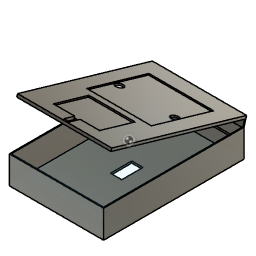
Round2-CAD (Autodesk Fusion 360 design; units mm, degrees)
Autodesk Fusion 360 part; units mm, degrees
sketch "Sketch6" plane through (0, 0, 0) normal (0, 0, 1) x (1, 0, 0)
  line L0 (0, 0) -> (0, 152)
  line L1 (0, 152) -> (102, 152)
  line L2 (102, 152) -> (102, 0)
  line L3 (102, 0) -> (0, 0)
  line L4 (375, 0) -> (375, 150)
  line L5 (375, 150) -> (475, 150)
  line L6 (475, 150) -> (475, 0)
  line L7 (475, 0) -> (375, 0)
  dimension "d16" = 152
  dimension "d17" = 102
  dimension "d89" = 150
  dimension "d90" = 100
  constraint coincident L0.start L3.end
  constraint vertical L0
  constraint perpendicular L0 L1
  constraint perpendicular L1 L2
  constraint perpendicular L0 L3
  constraint vertical L4
  constraint perpendicular L4 L5
  constraint perpendicular L5 L6
  constraint perpendicular L4 L7
  measures "d16" distance of L0.start L0.end
  measures "d17" distance of L0.end L1.end
  measures "d89" distance of L4.start L4.end
  measures "d90" distance of L4.end L5.end
extrude "Extrude2" add sketch "Sketch6" along normal blind 30 contours L0 L1 L2 L3 picked at (34, 101.333333)
shell "Shell1" thickness 2 removed faces 1 at (34, 101.333333, 30)
sketch "Sketch7" plane through (0, 0, 0) normal (0, 0, -1) x (1, 0, 0)
  line L0 (102, -152) -> (102, 0)
  line L1 (102, 0) -> (0, 0)
  line L2 (0, 0) -> (0, -152)
  line L3 (0, -152) -> (102, -152)
  line L4 (57.1, -64.5) -> (44.9, -64.5)
  line L5 (57.1, -87.5) -> (57.1, -64.5)
  line L6 (57.1, -64.5) -> (44.9, -64.5)
  line L7 (44.9, -64.5) -> (44.9, -87.5)
  line L8 (44.9, -87.5) -> (57.1, -87.5)
  line L9 (57.1, -87.5) -> (57.1, -64.5)
  constraint vertical L5
  constraint horizontal L6
  constraint vertical L7
  constraint horizontal L8
  constraint vertical L9
extrude "Extrude3" cut sketch "Sketch7" against normal blind 30 contours L4 L5 L6 L7 L8 L9 picked at (48.966667, -72.166667)
sketch "Sketch10" plane through (0, 0, 0) normal (-1, 0, 0) x (0, -1, 0)
  line L0 (-152, 0) -> (0, 0)
  line L1 (0, 0) -> (0, 30)
  line L2 (0, 30) -> (-152, 30)
  line L3 (-152, 30) -> (-152, 0)
  line L4 (-152, 30) -> (-6.038555, 72.417643)
  line L5 (-6.038555, 72.417643) -> (-5.201364, 69.536825)
  line L6 (-5.201364, 69.536825) -> (-151.16281, 27.119182)
  line L7 (-151.16281, 27.119182) -> (-152, 30)
  dimension "d30" = 152
  dimension "d31" = 3
  constraint perpendicular L4 L5
  constraint parallel L4 L6
  constraint parallel L5 L7
  constraint coincident L2.end L3.start
extrude "Extrude4" add sketch "Sketch10" against normal blind 102 contours L2 L4 L5 L6 picked at (-99.76277, 44.139214)
sketch "Sketch11" plane through (0, 19.876523, 68.396211) normal (0, 0.279063, 0.960273) x (-1, 0, 0)
  line L0 (0, -137.589542) -> (0, 14.410458)
  line L1 (0, 14.410458) -> (-102, 14.410458)
  line L2 (-102, 14.410458) -> (-102, -137.589542)
  line L3 (-102, -137.589542) -> (0, -137.589542)
  line L4 (-85.31414, -47.669713, 3.681927) -> (-15.31414, -47.669713, 3.681927)
  line L5 (-15.31414, -47.669713, 3.681927) -> (-15.31414, -117.669713, 3.681927)
  line L6 (-15.31414, -117.669713, 3.681927) -> (-85.31414, -117.669713, 3.681927)
  line L7 (-85.31414, -117.669713, 3.681927) -> (-85.31414, -47.669713, 3.681927)
  line L8 (-85.31414, -47.669713, 3.681927) -> (-15.31414, -117.669713, 3.681927) construction
  line L9 (-15.31414, -47.669713, 3.681927) -> (-85.31414, -117.669713, 3.681927) construction
  circle A0 centre (-80, -80) radius 3.5
  circle A1 centre (-20, -80) radius 3.5
  point P0 (-50.31414, -82.669713)
  dimension "d34" = 70
  dimension "d35" = 70
  dimension "d38" = 7
  dimension "d39" = 7
  measures "d38" diameter of A0
  measures "d39" diameter of A1
extrude "Extrude5" cut sketch "Sketch11" against normal blind 5 contours L4 L5 L6 L7 in plane through (0, 20.904007, 71.931839) normal (0, 0.27906344, 0.96027267) picked at (61.980806, 89.086291, 52.117485)
extrude "Extrude6" cut sketch "Sketch11" against normal blind 10 draft 30 contours A0 | A1 picked at (-81.114835, -79.656119) picked at (-20.259608, -78.862584)
sketch "Sketch12" plane through (0, 19.876523, 68.396211) normal (0, 0.279063, 0.960273) x (-1, 0, 0)
  line L0 (-15.31414, -47.669713) -> (-15.31414, -117.669713)
  line L1 (-15.31414, -117.669713) -> (-85.31414, -117.669713)
  line L2 (-85.31414, -117.669713) -> (-85.31414, -47.669713)
  line L3 (-85.31414, -47.669713) -> (-15.31414, -47.669713)
  line L4 (0, -137.589542) -> (0, 14.410458)
  line L5 (0, 14.410458) -> (-102, 14.410458)
  line L6 (-102, 14.410458) -> (-102, -137.589542)
  line L7 (-102, -137.589542) -> (0, -137.589542)
  line L8 (-50, 0) -> (-75, 0) construction
  line L9 (-75, 0) -> (-25, 0)
  line L10 (-25, 0) -> (-25, -40)
  line L11 (-25, -40) -> (-75, -40)
  line L12 (-75, -40) -> (-75, 0)
  dimension "d43" = 50
  dimension "d44" = 40
  constraint horizontal L9
  constraint vertical L10
  constraint horizontal L11
  constraint vertical L12
  measures "d43" distance of L8.end L9.end
  measures "d44" distance of L8.end L11.end
extrude "Extrude7" cut sketch "Sketch12" against normal blind 0.5 contours L9 L10 L11 L12 picked at (-58.333333, -13.333333)
extrude "Extrude8" cut 1 faces at (58.333333, 45.344263, 60.474383) along direction (0, -0.27906344, -0.96027267) blind 1
sketch "Sketch15" plane through (0, 19.876523, 68.396211) normal (0, 0.279063, 0.960273) x (-1, 0, 0)
  line L0 (-25, 0) -> (-25, -40)
  line L1 (-25, -40) -> (-75, -40)
  line L2 (-75, -40) -> (-75, 0)
  line L3 (-75, 0) -> (-25, 0)
  line L4 (-15.31414, -47.669713) -> (-15.31414, -117.669713)
  line L5 (-15.31414, -117.669713) -> (-85.31414, -117.669713)
  line L6 (-85.31414, -117.669713) -> (-85.31414, -47.669713)
  line L7 (-85.31414, -47.669713) -> (-15.31414, -47.669713)
  line L8 (0, -137.589542) -> (0, 14.410458)
  line L9 (0, 14.410458) -> (-102, 14.410458)
  line L10 (-102, 14.410458) -> (-102, -137.589542)
  line L11 (-102, -137.589542) -> (0, -137.589542)
  line L12 (-51, 0) -> (-54, 0)
  line L13 (-54, 0) -> (-48, 0)
  line L14 (-48, 0) -> (-48, 12)
  line L15 (-48, 12) -> (-54, 12)
  line L16 (-54, 12) -> (-54, 0)
  dimension "d49" = 3
  dimension "d50" = 6
  dimension "d51" = 12
  constraint coincident L3 L12.start
  constraint horizontal L13
  constraint vertical L14
  constraint horizontal L15
  constraint vertical L16
  measures "d49" distance of L12.start L12.end
  measures "d50" distance of L12.end L13.end
  measures "d51" distance of L12.end L15.end
extrude "Extrude9" cut sketch "Sketch15" against normal blind 10 contours L3 L12 L13 L14 L15 L16 picked at (-51, 8)
sketch "Sketch16" plane through (0, 0, 2) normal (0, 0, 1) x (-1, 0, 0)
  line L0 (-57.1, -64.5) -> (-44.9, -64.5)
  line L1 (-44.9, -64.5) -> (-44.9, -87.5)
  line L2 (-44.9, -87.5) -> (-57.1, -87.5)
  line L3 (-57.1, -87.5) -> (-57.1, -64.5)
  line L4 (-100, -2) -> (-100, -150)
  line L5 (-100, -150) -> (-2, -150)
  line L6 (-2, -150) -> (-2, -2)
  line L7 (-2, -2) -> (-100, -2)
extrude "Extrude13" cut 1 faces at (34.666667, 150, 11.333333) along direction (0, 1, 0) blind 1
extrude "Extrude14" cut 1 faces at (2, 98.083252, 11.333333) along direction (-1, 0, 0) blind 1
extrude "Extrude15" cut 1 faces at (100, 98.083252, 11.333333) along direction (1, 0, 0) blind 1
sketch "Sketch19" plane through (0, 151, 0) normal (0, -1, 0) x (1, 0, 0)
  line L0 (1, 2) -> (101, 2)
  line L1 (101, 2) -> (101, 30)
  line L2 (101, 30) -> (1, 30)
  line L3 (1, 30) -> (1, 2)
  line L4 (1, 2) -> (1, 17) construction
  line L5 (1, 17) -> (101, 17)
  line L6 (101, 17) -> (101, 16)
  line L7 (101, 16) -> (1, 16)
  line L8 (1, 16) -> (1, 17)
  dimension "d69" = 15
  dimension "d70" = 1
  constraint coincident L0.start L3.end
  constraint perpendicular L0 L4
  constraint horizontal L5
  constraint vertical L6
  constraint horizontal L7
  constraint vertical L8
  constraint coincident L1 L6.end
  measures "d69" distance of L0.start L4.end
  measures "d70" distance of L4.end L7.end
extrude "Extrude16" add sketch "Sketch19" along normal blind 1 contours L1 L3 L5 L6 L7 L8 picked at (34.333333, 16.666667)
sketch "Sketch20" plane through (0, 2, 0) normal (0, 1, 0) x (-1, 0, 0)
  line L0 (-101, 2) -> (-1, 2)
  line L1 (-1, 2) -> (-1, 30)
  line L2 (-1, 30) -> (-101, 30)
  line L3 (-101, 30) -> (-101, 2)
  line L4 (-1, 2) -> (-1, 17) construction
  line L5 (-1, 17) -> (-101, 17)
  line L6 (-101, 17) -> (-101, 18)
  line L7 (-101, 18) -> (-1, 18)
  line L8 (-1, 18) -> (-1, 17)
  dimension "d74" = 1
  constraint coincident L0.end L1.start
  constraint perpendicular L0 L4
  constraint horizontal L5
  constraint vertical L6
  constraint horizontal L7
  constraint vertical L8
  constraint coincident L3 L6.end
  measures "d74" distance of L4.end L7.end
extrude "Extrude17" add sketch "Sketch20" along normal blind 1 contours L1 L3 L5 L6 L7 L8 picked at (-67.666667, 17.666667)
extrude "Extrude18" cut 1 faces at (67.666667, 2, 7) along direction (0, -1, 0) blind 1
extrude "Extrude19" cut 1 faces at (67.666667, 2, 22) along direction (0, -1, 0) blind 1
extrude "Extrude20" add 1 faces at (67.666667, 1, 7) along direction (0, 1, 0) blind 2
extrude "Extrude21" add 1 faces at (67.666667, 151, 11.333333) along direction (0, -1, 0) blind 2
extrude "Extrude22" cut 1 faces at (67.666667, 149, 11.333333) along direction (0, 1, 0) blind 1
extrude "Extrude23" add 1 faces at (34.333333, 150, 12) along direction (0, -1, 0) blind 1
sketch "Sketch21" plane through (0, 0, 2) normal (0, 0, 1) x (-1, 0, 0)
extrude "Extrude24" add 1 faces at (87.438047, 30.522508, 65.302397) along direction (0, 0.27906344, 0.96027267) blind 10
extrude "Extrude25" add 1 faces at (59.168247, 121.373661, 37.527645) along direction (0, 0.27906344, 0.96027267) blind 10
extrude "Extrude26" add 1 faces at (49.333333, 45.065199, 59.51411) along direction (0, 0.27906344, 0.96027267) blind 10
extrude "Extrude27" cut 1 faces at (49.333333, 67.635159, 51.393031) along direction (0, 0.27906344, 0.96027267) blind 10
delete_face "DeleteFace1" 1 faces at (84.5949, 99.194199, 45.69294)
delete_face "DeleteFace2" 1 faces at (14.793948, 97.221321, 49.737512)
extrude "Extrude28" cut 1 faces at (67.666667, 143.110179, 36.401818) along direction (0, 0.96027267, -0.27906344) blind 5
extrude "Extrude29" cut 1 faces at (67.666667, 148.046706, 35.471606) along direction (0, 0.96027267, -0.27906344) blind 4
delete_face "DeleteFace3" 1 faces at (0.333333, 147.011392, 28.325619)
delete_face "DeleteFace4" 1 faces at (101.333333, 147.011392, 28.325619)
sketch "Sketch22" plane through (0, 1, 0) normal (0, 1, 0) x (-1, 0, 0)
  line L0 (-101, 18) -> (-1, 18)
  line L1 (-1, 18) -> (-1, 30)
  line L2 (-1, 30) -> (-101, 30)
  line L3 (-101, 30) -> (-101, 18)
extrude "Extrude10" [suppressed]
extrude "Extrude11" [suppressed]
extrude "Extrude12" [suppressed]
